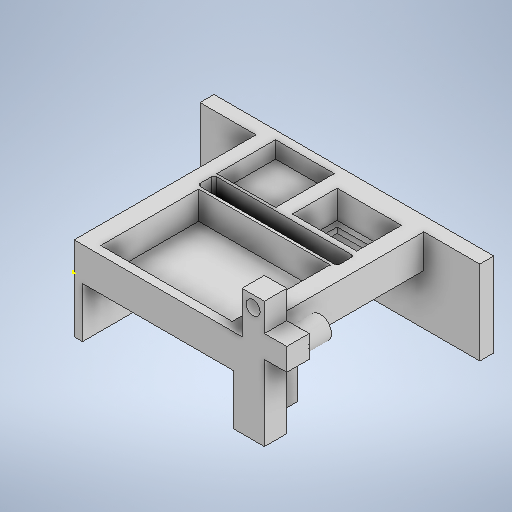
# Autodesk Inventor part: Platform
Saved by Autodesk Inventor 2025.2 (Build 292293000, 293)
## iProperties
Created: 2026-01-09
Part Number: Platform
Material: Generic
Document SubType Name: Modeling
Designer: William
Density: 1 g/cm^3
Appearance: Default
Author: William
Autodesk Inventor part; units mm, degrees
ref_plane "YZ Plane" through (0, 0, 0) normal (1, 0, 0) x (0, 1, 0)
ref_plane "XZ Plane" through (0, 0, 0) normal (0, 1, 0) x (-1, 0, 0)
sketch "Sketch1" plane through (0, 0, 0) normal (0, 1, 0) x (-1, 0, 0)
  line L0 (0, 0) -> (-60, 0)
  line L1 (-60, 0) -> (-60, -70)
  line L2 (-60, -70) -> (0, -70)
  line L3 (0, -70) -> (0, 0)
  dimension "d0" = 60
  dimension "d1" = 70
  constraints: 8 end point, 2 parallel, 1 horizontal, 1 perpendicular
  measures "d0" distance of L2.end L1.end
  measures "d1" distance of L1.end L0.end
extrude "Extrusion1" add sketch "Sketch1" along normal blind 12
sketch "Sketch2" plane through (0, 0, 0) normal (0, -1, 0) x (1, 0, 0)
  line L0 (60, -70) -> (0, -70) projected
  line L1 (60, 0) -> (60, -70) projected
  line L2 (0, -70) -> (60, -70)
  line L3 (60, -70) -> (60, -65)
  line L4 (60, -65) -> (0, -65)
  line L5 (0, -65) -> (0, -70)
  line L6 (60, 0) -> (57, 0)
  line L7 (57, 0) -> (57, -20)
  line L8 (57, -20) -> (60, -20)
  line L9 (60, -20) -> (60, 0)
  line L10 (0, -70) -> (0, 0) projected
  line L11 (0, 0) -> (3, 0)
  line L12 (3, 0) -> (3, -20)
  line L13 (3, -20) -> (0, -20)
  line L14 (0, -20) -> (0, 0)
  point P0 (0, -20)
  dimension "d4" = 5
  dimension "d9" = 3
  dimension "d10" = 20
  dimension "d11" = 3
  dimension "d12" = 20
  constraints: 24 end point, 6 parallel, 3 horizontal, 3 perpendicular, 1 point on line
  measures "d4" distance of L3.end L2.end
  measures "d9" distance of L8.end L7.end
  measures "d10" distance of L7.end L6.end
  measures "d11" distance of L12.end L13.end
  measures "d12" distance of L11.end L12.end
extrude "Extrusion2" add sketch "Sketch2" along normal blind 18
sketch "Sketch3" plane through (60, 0, 0) normal (1, 0, 0) x (0, 0, -1)
  line L0 (65, 0) -> (65, -18) projected
  line L1 (70, -18) -> (70, 12) projected
  line L2 (65, -18) -> (70, -18)
  line L3 (70, -18) -> (70, 12)
  line L4 (70, 12) -> (65, 12)
  line L5 (65, 12) -> (65, -18)
  point P0 (0, 0)
  constraints: 8 end point, 2 parallel, 1 horizontal, 1 perpendicular
extrude "Extrusion3" add sketch "Sketch3" along normal blind 20
ref_plane "Work Plane1" through (30, 0, 0) normal (1, 0, 0) x (0, 0, -1)
mirror "Mirror1" about plane through (30, 0, 0) normal (1, 0, 0) of "Extrusion3"
sketch "Sketch4" plane through (0, 12, 0) normal (0, 1, 0) x (1, 0, 0)
  line L0 (6.5, 38) -> (53.5, 38)
  line L1 (53.5, 38) -> (53.5, 3)
  line L2 (53.5, 3) -> (6.5, 3)
  line L3 (6.5, 3) -> (6.5, 38)
  line L4 (5, 67) -> (26, 67)
  line L5 (26, 67) -> (26, 46)
  line L6 (26, 46) -> (5, 46)
  line L7 (5, 46) -> (5, 67)
  line L8 (31, 63) -> (54, 63)
  line L9 (54, 63) -> (54, 47)
  line L10 (54, 47) -> (31, 47)
  line L11 (31, 47) -> (31, 63)
  line L12 (0, 0) -> (60, 0) projected
  line L13 (-20, 70) -> (80, 70) projected
  line L14 (0, 65) -> (0, 0) projected
  line L15 (60, 0) -> (60, 65) projected
  point P0 (30, 38)
  point P1 (30, 0)
  dimension "d13" = 47
  dimension "d14" = 35
  dimension "d15" = 21
  dimension "d16" = 21
  dimension "d17" = 23
  dimension "d18" = 16
  dimension "d19" = 3
  dimension "d20" = 7
  dimension "d21" = 3
  dimension "d30" = 5
  dimension "d31" = 6
  constraints: 24 end point, 6 parallel, 3 horizontal, 3 perpendicular, 2 midpoint, 1 vertical alignment
  measures "d13" distance of L1.end L2.end
  measures "d14" distance of L0.end L1.end
  measures "d15" distance of L5.end L6.end
  measures "d16" distance of L4.end L5.end
  measures "d17" distance of L9.end L10.end
  measures "d18" distance of L8.end L9.end
  measures "d19" distance between parallel lines of L12 L2
  measures "d20" distance between parallel lines of L13 L8
  measures "d21" distance between parallel lines of L13 L4
  measures "d30" distance between parallel lines of L14 L7
  measures "d31" distance between parallel lines of L15 L9
sketch "Sketch5" plane through (0, 12, 0) normal (0, 1, 0) x (1, 0, 0)
  line L0 (54, 45) -> (6, 45)
  line L1 (5, 44) -> (5, 40)
  line L2 (6, 39) -> (54, 39)
  line L3 (55, 40) -> (55, 44)
  line L4 (26, 46) -> (5, 46) projected
  line L5 (-20, 70) -> (80, 70) projected
  line L6 (0, 65) -> (0, 0) projected
  arc A0 (54, 39) -> (55, 40) centre (54, 40) ccw
  arc A1 (55, 44) -> (54, 45) centre (54, 44) ccw
  arc A2 (6, 45) -> (5, 44) centre (6, 44) ccw
  arc A3 (5, 40) -> (6, 39) centre (6, 40) ccw
  point P0 (55, 45)
  point P1 (5, 39)
  point P2 (55, 39)
  dimension "d22" = 50
  dimension "d23" = 25
  dimension "d24" = 6
  dimension "d25" = 5
  dimension "d26" = 1
  dimension "d27" = 1
  constraints: 8 end point, 8 point on circle, 8 tangent, 6 point on line, 4 centre point, 2 equal radius, 2 parallel, 1 horizontal, 1 perpendicular
  measures "d22" distance of point (55, 39) point (5, 39)
  measures "d23" distance between parallel lines of L5 L0
  measures "d24" distance of point (55, 39) point (55, 45)
  measures "d25" distance between parallel lines of L6 L1
  measures "d26" radius of A0
  measures "d27" radius of A1
extrude "Extrusion4" cut sketch "Sketch5" against normal blind 25
extrude "Extrusion5" cut sketch "Sketch4" against normal blind 10
sketch "Sketch6" plane through (0, 2, 0) normal (0, 1, 0) x (1, 0, 0)
  line L0 (54, 47) -> (31, 47) projected
  line L1 (54, 63) -> (54, 47) projected
  line L2 (31, 63) -> (54, 63) projected
  line L3 (31, 47) -> (31, 63) projected
  line L4 (33, 61) -> (52, 61)
  line L5 (52, 61) -> (52, 49)
  line L6 (52, 49) -> (33, 49)
  line L7 (33, 49) -> (33, 61)
  point P0 (0, 0)
  dimension "d34" = 2
  constraints: 8 end point, 3 other
  measures "d34" distance between parallel lines of L3 L7
extrude "Extrusion6" cut sketch "Sketch6" against normal blind 12 contours L4 L5 L6 L7
sketch "Sketch7" plane through (0, 2, 0) normal (0, 1, 0) x (1, 0, 0)
  point P0 (0, 0)
sketch "Sketch8" plane through (0, 2, 0) normal (0, 1, 0) x (1, 0, 0)
  line L0 (26, 46) -> (5, 46) projected
  line L1 (26, 67) -> (26, 46) projected
  line L2 (5, 67) -> (26, 67) projected
  line L3 (5, 46) -> (5, 67) projected
  point P0 (0, 0)
extrude "Extrusion7" add sketch "Sketch8" along normal blind 4
sketch "Sketch9" plane through (60, 0, -20) normal (1, 0, 0) x (0, 0, -1)
  line L0 (-20, 12) -> (-20, -18) projected
  line L1 (-20, -18) -> (-12, -18)
  line L2 (-12, -18) -> (-12, 27)
  line L3 (-12, 27) -> (-20, 27)
  line L4 (-20, 27) -> (-20, -18)
  point P0 (-20, 0)
  dimension "d39" = 8
  dimension "d40" = 45
  constraints: 8 end point, 2 parallel, 1 horizontal, 1 perpendicular
  measures "d39" distance of L3.end L2.end
  measures "d40" distance of L2.end L1.end
extrude "Extrusion8" add sketch "Sketch9" along normal blind 8
sketch "Sketch10" plane through (3, 0, 0) normal (0, 0, 1) x (1, 0, 0)
  circle A0 centre (61, 23) radius 2.5
  line L0 (57, 27) -> (65, 27) projected
  point P0 (-3, 0)
  point P1 (61, 27)
  dimension "d43" = 5
  dimension "d44" = 4
  constraints: 1 centre point, 1 midpoint
  measures "d43" diameter of A0
  measures "d44" distance of A0.centre point (61, 27)
extrude "Extrusion9" cut sketch "Sketch10" against normal blind 10
sketch "Sketch12" plane through (68, 0, -20) normal (1, 0, 0) x (0, 0, -1)
  line L0 (-20, 27) -> (-20, -18) projected
  line L1 (-12, 12) -> (-12, -18) projected
  line L2 (-20, 17) -> (-12, 17)
  line L3 (-12, 17) -> (-12, 9)
  line L4 (-12, 9) -> (-20, 9)
  line L5 (-20, 9) -> (-20, 17)
  line L6 (-12, 27) -> (-20, 27) projected
  point P0 (-20, 0)
  dimension "d47" = 10
  dimension "d48" = 8
  constraints: 8 end point, 2 parallel, 2 point on line, 1 horizontal, 1 perpendicular
  measures "d47" distance between parallel lines of L6 L2
  measures "d48" distance between parallel lines of L2 L4
extrude "Extrusion10" add sketch "Sketch12" along normal blind 8
sketch "Sketch13" plane through (60, 12, -8) normal (0, 0, -1) x (-1, 0, 0)
  circle A0 centre (-12, 1) radius 4
  line L0 (-8, 5) -> (-16, 5) projected
  line L1 (-16, -3) -> (-16, 5) projected
  point P0 (60, -12)
  dimension "d51" = 8
  constraints: 2 tangent, 1 centre point
  measures "d51" diameter of A0
extrude "Extrusion11" add sketch "Sketch13" along normal blind 8 contours A0
body "Solid1"
